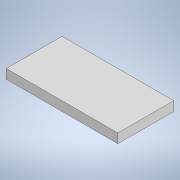
# Autodesk Inventor part: peg toy side
Saved by Autodesk Inventor 2021 (Build 250183000, 183)
## iProperties
Created: 2020-12-18
Part Number: peg toy side
Material: Generic
Document SubType Name: Modeling
Designer: Jawad
Density: 1 g/cm^3
Appearance: Default
Author: Jawad
Autodesk Inventor part; units mm, degrees
ref_plane "YZ Plane" through (0, 0, 0) normal (1, 0, 0) x (0, 1, 0)
ref_plane "XZ Plane" through (0, 0, 0) normal (0, 1, 0) x (-1, 0, 0)
ref_plane "XY Plane" through (0, 0, 0) normal (0, 0, 1) x (1, 0, 0)
sketch "Sketch1" plane through (0, 0, 0) normal (0, 1, 0) x (-1, 0, 0)
  line L0 (18.4943, 21.0728) -> (-133.9057, 21.0728)
  line L1 (-133.9057, 21.0728) -> (-133.9057, -55.1272)
  line L2 (-133.9057, -55.1272) -> (18.4943, -55.1272)
  line L3 (18.4943, -55.1272) -> (18.4943, 21.0728)
  point P0 (0, 0)
  dimension "d0" = 76.2
  dimension "d1" = 152.4
  constraints: 8 end point, 2 parallel, 1 horizontal, 1 perpendicular
  measures "d0" distance of L2.end L0.start
  measures "d1" distance of L1.end L2.end
extrude "Extrusion1" add sketch "Sketch1" along normal blind 12.7
body "Solid1"
